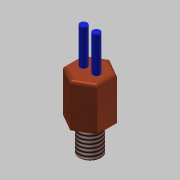
# Autodesk Inventor part: Part20
Saved by Autodesk Inventor 2014 (Build 180170000, 170)
## iProperties
Created: 2016-04-22
Part Number: Part20
Material: Copper
Document SubType Name: Modeling
Designer: admin
Density: 8.94 g/cm^3
Appearance: Copper - Satin
Author: admin
Autodesk Inventor part; units mm, degrees
ref_plane "YZ Plane" through (0, 0, 0) normal (1, 0, 0) x (0, 1, 0)
ref_plane "XZ Plane" through (0, 0, 0) normal (0, 1, 0) x (-1, 0, 0)
ref_plane "XY Plane" through (0, 0, 0) normal (0, 0, 1) x (1, 0, 0)
sketch "Sketch1" plane through (0, 0, 0) normal (0, 0, 1) x (1, 0, 0)
  circle A0 centre (8, 4) radius 1.2295 projected
  circle A1 centre (-1.5, 4) radius 3 projected
  line L0 (10, 0) -> (-5.5, 0) projected
  line L1 (10, 0) -> (10, 10) projected
  line L2 (10, 10) -> (-5.5, 10) projected
  line L3 (-5.5, 0) -> (-5.5, 10) projected
  line L4 (10.4, 2.6144) -> (8, 1.2287)
  line L5 (8, 1.2287) -> (5.6, 2.6144)
  line L6 (5.6, 2.6144) -> (5.6, 5.3856)
  line L7 (5.6, 5.3856) -> (8, 6.7713)
  line L8 (8, 6.7713) -> (10.4, 5.3856)
  line L9 (10.4, 5.3856) -> (10.4, 2.6144)
  point P0 (0, 0)
  dimension "d0" = 2.4
  constraints: 12 end point, 1 coincident, 1 parallel, 13 other
  measures "d0" distance from line of L9 A0.centre
extrude "Extrusion1" add sketch "Sketch1" along normal blind 6 contours A0 | L4 L5 L6 L7 L8 L1 | L1 L8 L9 L4
fillet "Fillet1" radius 0.5 6 edges at (10.4, 4, 6) (9.2, 6.0785, 6) (6.8, 6.0785, 6) (5.6, 4, 6) (6.8, 1.9215, 6) (9.2, 1.9215, 6)
sketch "Sketch2" plane through (0, 0, 6) normal (0, 0, 1) x (1, 0, 0)
  line L0 (6.1, 2.903) -> (6.1, 5.097) projected
  line L1 (9.9, 5.097) -> (9.9, 2.903) projected
  circle A0 centre (7.1, 4) radius 0.5
  circle A1 centre (8.9, 4) radius 0.5
  point P0 (0, 0)
  dimension "d4" = 1
  dimension "d5" = 1
  dimension "d6" = 1
  dimension "d7" = 1
  constraints: 2 centre point
  measures "d4" diameter of A0
  measures "d5" diameter of A1
  measures "d6" distance from line of L0 A0.centre
  measures "d7" distance from line of L1 A1.centre
extrude "Extrusion2" add sketch "Sketch2" along normal blind 5 separate body
sketch "Sketch3" plane through (0, 0, 0) normal (0, 0, -1) x (-1, 0, 0)
  circle A0 centre (-8, 4) radius 1.5
  point P0 (0, 0)
  dimension "d10" = 3
  constraints: 1 centre point
  measures "d10" diameter of A0
extrude "Extrusion3" add sketch "Sketch3" along normal blind 4 bodies 1
thread "Thread1" size "M3x0.5" class "6g" standard "ANSI Metric M Profile" full length
body "Solid1"
body "Solid2"
